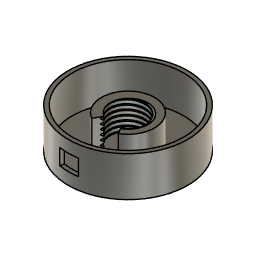
BottomPlate v3 (Autodesk Fusion 360 design; units mm, degrees)
Autodesk Fusion 360 part; units mm, degrees
sketch "Sketch1" plane through (0, 0, 0) normal (0, 0, 1) x (1, 0, 0)
sketch "Sketch2" plane through (0, 0, 0) normal (0, 0, 1) x (1, 0, 0)
  circle A0 centre (0, 0) radius 45
  dimension "d1" = 90
  constraint coincident A0.centre origin
  measures "d1" diameter of A0
extrude "Extrude1" add sketch "Sketch2" along normal blind 2
sketch "Sketch3" plane through (0, 0, 2) normal (0, 0, 1) x (-1, 0, 0)
  circle A0 centre (0, 0) radius 45
  circle A1 centre (0, 0) radius 42
  dimension "d4" = 84
  constraint concentric A0 A1
  measures "d4" diameter of A1
extrude "Extrude2" add sketch "Sketch3" along normal blind 28
sketch "Sketch4" plane through (0, 0, 0) normal (1, 0, 0) x (0, 1, 0)
  line L0 (15, 2) -> (20, 2)
  line L1 (20, 2) -> (20, 25)
  line L2 (20, 25) -> (15, 25)
  line L3 (15, 25) -> (15, 2)
  constraint horizontal L0
  constraint vertical L1
  constraint horizontal L2
  constraint vertical L3
revolve "Revolve1" add sketch "Sketch4" angle 150 about axis through (0, 0, 1.75) along (0, 0, -1) second angle 150
thread "Thread1" "ISO Metric profile 30.0 M30x3.5 6H" major diameter 30.3925 minor diameter 26.491 pitch 3.5 angle 60 modelled right hand crest width 0.9556 on face at (8.7562, -12.1791, 17.3333) crest through (0, 13.2455, 24.125)
sketch "Sketch5" plane through (0, 0, 0) normal (1, 0, 0) x (0, 1, 0)
  line L0 (-45, 9) -> (-42, 9)
  line L1 (-42, 9) -> (-42, 21)
  line L2 (-42, 21) -> (-45, 21)
  line L3 (-45, 21) -> (-45, 9)
  constraint horizontal L0
  constraint vertical L1
  constraint horizontal L2
  constraint vertical L3
revolve "Revolve2" cut sketch "Sketch5" angle 9 about axis through (0, 0, 1.75) along (0, 0, 1) second angle 9
